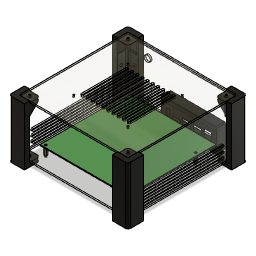
tp2_case_v1 (Autodesk Fusion 360 design; units mm, degrees)
Autodesk Fusion 360 part; units mm, degrees
sketch "Mini-ITX Board" plane through (0, 0, 0) normal (0, 1, 0) x (1, 0, 0)
  line L0 (0, 0) -> (170, 0)
  line L1 (170, 0) -> (170, 170)
  line L2 (170, 170) -> (0, 170)
  line L3 (0, 170) -> (0, 0)
  circle A0 centre (6.35, 159.84) radius 1.98
  circle A1 centre (6.35, 4.9) radius 1.98
  circle A2 centre (163.83, 4.9) radius 1.98
  circle A3 centre (163.83, 136.98) radius 1.98
  dimension "d1" = 170
  dimension "d2" = 170
  dimension "d3" = 3.96
  dimension "d4" = 10.16
  dimension "d5" = 6.35
  dimension "d6" = 3.96
  dimension "d7" = 154.94
  dimension "d8" = 6.35
  dimension "d9" = 3.96
  dimension "d10" = 157.48
  dimension "d11" = 154.94
  dimension "d12" = 3.96
  dimension "d13" = 22.86
  dimension "d14" = 157.48
  constraint horizontal L0
  constraint vertical L1
  constraint horizontal L2
  constraint vertical L3
  constraint coincident L0.start L3.end
  measures "d1" distance of L0.start L0.end
  measures "d2" distance of L0.start L2.end
  measures "d3" diameter of A0
  measures "d4" distance of L2 A0.centre
  measures "d5" distance of L3 A0.centre
  measures "d6" diameter of A1
  measures "d7" vertical distance of A0.centre A1.centre
  measures "d8" distance of L3 A1.centre
  measures "d9" diameter of A2
  measures "d10" horizontal distance of A1.centre A2.centre
  measures "d11" vertical distance of A0.centre A2.centre
  measures "d12" diameter of A3
  measures "d13" vertical distance of A0.centre A3.centre
  measures "d14" horizontal distance of A1.centre A3.centre
sketch "Base" plane through (0, 0, 0) normal (0, 1, 0) x (1, 0, 0)
  line L0 (-17, -20) -> (187, -20)
  line L1 (190, -17) -> (190, 187)
  line L2 (187, 190) -> (-17, 190)
  line L3 (-20, 187) -> (-20, -17)
  line L4 (170, 170) -> (0, 170)
  line L5 (0, 0) -> (170, 0)
  line L6 (170, 0) -> (170, 170)
  line L7 (0, 170) -> (0, 0)
  circle A0 centre (6.35, 159.84) radius 1.6
  circle A1 centre (6.35, 4.9) radius 1.6
  circle A2 centre (163.83, 4.9) radius 1.6
  circle A3 centre (163.83, 136.98) radius 1.6
  arc A4 (-17, 190) -> (-20, 187) centre (-17, 187) ccw
  arc A5 (190, 187) -> (187, 190) centre (187, 187) ccw
  arc A6 (187, -20) -> (190, -17) centre (187, -17) ccw
  arc A7 (-20, -17) -> (-17, -20) centre (-17, -17) ccw
  circle A8 centre (-10, -10) radius 1.6
  circle A9 centre (180, -10) radius 1.6
  circle A10 centre (180, 180) radius 1.6
  circle A11 centre (-10, 180) radius 1.6
  point P0 (6.35, 159.84)
  point P1 (163.83, 136.98)
  point P2 (163.83, 4.9)
  point P3 (6.35, 4.9)
  dimension "d15" = 20
  dimension "d16" = 20
  dimension "d17" = 20
  dimension "d18" = 20
  dimension "d19" = 3.2
  dimension "d20" = 3.2
  dimension "d21" = 3.2
  dimension "d22" = 3.2
  dimension "d57" = 3
  dimension "d88" = 3.2
  dimension "d89" = 10
  dimension "d90" = 10
  dimension "d91" = 3.2
  dimension "d92" = 10
  dimension "d93" = 10
  dimension "d94" = 3.2
  dimension "d95" = 10
  dimension "d96" = 10
  dimension "d97" = 3.2
  dimension "d98" = 10
  dimension "d99" = 10
  constraint horizontal L0
  constraint vertical L1
  constraint horizontal L2
  constraint vertical L3
  constraint coincident P0 A0.centre
  constraint coincident P3 A1.centre
  constraint coincident P2 A2.centre
  constraint coincident P1 A3.centre
  constraint tangent L2 A4
  constraint tangent L3 A4
  constraint tangent L1 A5
  constraint tangent L2 A5
  constraint equal A4 A5
  constraint tangent L0 A6
  constraint tangent L1 A6
  constraint equal A4 A6
  constraint tangent L0 A7
  constraint tangent L3 A7
  constraint equal A4 A7
  measures "d15" distance of L2 L4
  measures "d16" distance of L0 L5
  measures "d17" distance of L1 L6
  measures "d18" distance of L3 L7
  measures "d19" diameter of A0
  measures "d20" diameter of A1
  measures "d21" diameter of A2
  measures "d22" diameter of A3
  measures "d57" radius of A4
  measures "d88" diameter of A8
  measures "d89" distance of L0 A8.centre
  measures "d90" distance of L3 A8.centre
  measures "d91" diameter of A9
  measures "d92" distance of L1 A9.centre
  measures "d93" distance of L0 A9.centre
  measures "d94" diameter of A10
  measures "d95" distance of L1 A10.centre
  measures "d96" distance of L2 A10.centre
  measures "d97" diameter of A11
  measures "d98" distance of L2 A11.centre
  measures "d99" distance of L3 A11.centre
sketch "Top" plane through (0, 0, 0) normal (0, 1, 0) x (1, 0, 0)
  line L0 (-17, 190) -> (187, 190)
  line L1 (190, 187) -> (190, -17)
  line L2 (187, -20) -> (-17, -20)
  line L3 (-20, -17) -> (-20, 187)
  arc A0 (-17, 190) -> (-20, 187) centre (-17, 187) ccw
  arc A1 (190, 187) -> (187, 190) centre (187, 187) ccw
  arc A2 (187, -20) -> (190, -17) centre (187, -17) ccw
  arc A3 (-20, -17) -> (-17, -20) centre (-17, -17) ccw
  circle A4 centre (-10, -10) radius 1.6
  circle A5 centre (180, -10) radius 1.6
  circle A6 centre (180, 180) radius 1.6
  circle A7 centre (-10, 180) radius 1.6
  circle A8 centre (32.5, 137.5) radius 1.6
  circle A9 centre (137.5, 137.5) radius 1.6
  circle A10 centre (32.5, 32.5) radius 1.6
  circle A11 centre (137.5, 32.5) radius 1.6
  line L4 (35, 135) -> (135, 135)
  line L5 (135, 135) -> (135, 35)
  line L6 (135, 35) -> (35, 35)
  line L7 (35, 35) -> (35, 135)
  line L8 (39.5, 130) -> (40.5, 130)
  line L9 (42.5, 128) -> (42.5, 42)
  line L10 (40.5, 40) -> (39.5, 40)
  line L11 (37.5, 42) -> (37.5, 128)
  line L12 (49.5, 130) -> (50.5, 130)
  line L13 (52.5, 128) -> (52.5, 42)
  line L14 (47.5, 42) -> (47.5, 128)
  line L15 (50.5, 40) -> (49.5, 40)
  line L16 (59.5, 130) -> (60.5, 130)
  line L17 (62.5, 128) -> (62.5, 42)
  line L18 (57.5, 42) -> (57.5, 128)
  line L19 (60.5, 40) -> (59.5, 40)
  line L20 (69.5, 130) -> (70.5, 130)
  line L21 (72.5, 128) -> (72.5, 42)
  line L22 (67.5, 42) -> (67.5, 128)
  line L23 (70.5, 40) -> (69.5, 40)
  line L24 (79.5, 130) -> (80.5, 130)
  line L25 (82.5, 128) -> (82.5, 42)
  line L26 (77.5, 42) -> (77.5, 128)
  line L27 (80.5, 40) -> (79.5, 40)
  line L28 (89.5, 130) -> (90.5, 130)
  line L29 (92.5, 128) -> (92.5, 42)
  line L30 (87.5, 42) -> (87.5, 128)
  line L31 (90.5, 40) -> (89.5, 40)
  line L32 (99.5, 130) -> (100.5, 130)
  line L33 (102.5, 128) -> (102.5, 42)
  line L34 (97.5, 42) -> (97.5, 128)
  line L35 (100.5, 40) -> (99.5, 40)
  line L36 (109.5, 130) -> (110.5, 130)
  line L37 (112.5, 128) -> (112.5, 42)
  line L38 (107.5, 42) -> (107.5, 128)
  line L39 (110.5, 40) -> (109.5, 40)
  line L40 (119.5, 130) -> (120.5, 130)
  line L41 (122.5, 128) -> (122.5, 42)
  line L42 (117.5, 42) -> (117.5, 128)
  line L43 (120.5, 40) -> (119.5, 40)
  line L44 (129.5, 130) -> (130.5, 130)
  line L45 (132.5, 128) -> (132.5, 42)
  line L46 (127.5, 42) -> (127.5, 128)
  line L47 (130.5, 40) -> (129.5, 40)
  arc A12 (39.5, 130) -> (37.5, 128) centre (39.5, 128) ccw
  arc A13 (42.5, 128) -> (40.5, 130) centre (40.5, 128) ccw
  arc A14 (37.5, 42) -> (39.5, 40) centre (39.5, 42) ccw
  arc A15 (40.5, 40) -> (42.5, 42) centre (40.5, 42) ccw
  arc A16 (47.5, 42) -> (49.5, 40) centre (49.5, 42) ccw
  arc A17 (50.5, 40) -> (52.5, 42) centre (50.5, 42) ccw
  arc A18 (49.5, 130) -> (47.5, 128) centre (49.5, 128) ccw
  arc A19 (52.5, 128) -> (50.5, 130) centre (50.5, 128) ccw
  arc A20 (57.5, 42) -> (59.5, 40) centre (59.5, 42) ccw
  arc A21 (60.5, 40) -> (62.5, 42) centre (60.5, 42) ccw
  arc A22 (59.5, 130) -> (57.5, 128) centre (59.5, 128) ccw
  arc A23 (62.5, 128) -> (60.5, 130) centre (60.5, 128) ccw
  arc A24 (69.5, 130) -> (67.5, 128) centre (69.5, 128) ccw
  arc A25 (72.5, 128) -> (70.5, 130) centre (70.5, 128) ccw
  arc A26 (67.5, 42) -> (69.5, 40) centre (69.5, 42) ccw
  arc A27 (70.5, 40) -> (72.5, 42) centre (70.5, 42) ccw
  arc A28 (77.5, 42) -> (79.5, 40) centre (79.5, 42) ccw
  arc A29 (80.5, 40) -> (82.5, 42) centre (80.5, 42) ccw
  arc A30 (82.5, 128) -> (80.5, 130) centre (80.5, 128) ccw
  arc A31 (79.5, 130) -> (77.5, 128) centre (79.5, 128) ccw
  arc A32 (89.5, 130) -> (87.5, 128) centre (89.5, 128) ccw
  arc A33 (92.5, 128) -> (90.5, 130) centre (90.5, 128) ccw
  arc A34 (87.5, 42) -> (89.5, 40) centre (89.5, 42) ccw
  arc A35 (90.5, 40) -> (92.5, 42) centre (90.5, 42) ccw
  arc A36 (97.5, 42) -> (99.5, 40) centre (99.5, 42) ccw
  arc A37 (100.5, 40) -> (102.5, 42) centre (100.5, 42) ccw
  arc A38 (102.5, 128) -> (100.5, 130) centre (100.5, 128) ccw
  arc A39 (99.5, 130) -> (97.5, 128) centre (99.5, 128) ccw
  arc A40 (109.5, 130) -> (107.5, 128) centre (109.5, 128) ccw
  arc A41 (112.5, 128) -> (110.5, 130) centre (110.5, 128) ccw
  arc A42 (107.5, 42) -> (109.5, 40) centre (109.5, 42) ccw
  arc A43 (110.5, 40) -> (112.5, 42) centre (110.5, 42) ccw
  arc A44 (117.5, 42) -> (119.5, 40) centre (119.5, 42) ccw
  arc A45 (120.5, 40) -> (122.5, 42) centre (120.5, 42) ccw
  arc A46 (122.5, 128) -> (120.5, 130) centre (120.5, 128) ccw
  arc A47 (119.5, 130) -> (117.5, 128) centre (119.5, 128) ccw
  arc A48 (129.5, 130) -> (127.5, 128) centre (129.5, 128) ccw
  arc A49 (132.5, 128) -> (130.5, 130) centre (130.5, 128) ccw
  arc A50 (130.5, 40) -> (132.5, 42) centre (130.5, 42) ccw
  arc A51 (127.5, 42) -> (129.5, 40) centre (129.5, 42) ccw
  point P0 (-20, 190)
  point P1 (190, -20)
  point P2 (37.5, 130)
  point P3 (42.5, 130)
  point P4 (37.5, 40)
  dimension "d59" = 3
  dimension "d146" = 3.2
  dimension "d147" = 3.2
  dimension "d148" = 3.2
  dimension "d149" = 3.2
  dimension "d150" = 52.5
  dimension "d151" = 52.5
  dimension "d152" = 52.5
  dimension "d153" = 52.5
  dimension "d154" = 52.5
  dimension "d155" = 52.5
  dimension "d156" = 105
  dimension "d157" = 52.5
  dimension "d158" = 52.5
  dimension "d159" = 105
  dimension "d160" = 100
  dimension "d161" = 100
  dimension "d162" = 2.5
  dimension "d163" = 2.5
  dimension "d164" = 5
  dimension "d165" = 90
  dimension "d166" = 2.5
  dimension "d167" = 5
  dimension "d172" = 2
  constraint horizontal L0
  constraint vertical L1
  constraint horizontal L2
  constraint vertical L3
  constraint tangent L0 A0
  constraint tangent L3 A0
  constraint tangent L0 A1
  constraint tangent L1 A1
  constraint equal A0 A1
  constraint tangent L1 A2
  constraint tangent L2 A2
  constraint equal A0 A2
  constraint tangent L2 A3
  constraint tangent L3 A3
  constraint equal A0 A3
  constraint horizontal L4
  constraint vertical L5
  constraint horizontal L6
  constraint vertical L7
  constraint horizontal L8
  constraint vertical L9
  constraint horizontal L10
  constraint vertical L11
  constraint coincident P2 L8
  constraint coincident P2 L11
  constraint tangent L8 A12
  constraint tangent L11 A12
  constraint coincident P3 L8
  constraint coincident P3 L9
  constraint tangent L8 A13
  constraint tangent L9 A13
  constraint equal A12 A13
  constraint coincident P4 L10
  constraint coincident P4 L11
  constraint tangent L10 A14
  constraint tangent L11 A14
  constraint equal A12 A14
  constraint tangent L9 A15
  constraint tangent L10 A15
  constraint equal A12 A15
  constraint tangent L14 A16
  constraint tangent L15 A16
  constraint equal A12 A16
  constraint tangent L13 A17
  constraint tangent L15 A17
  constraint equal A12 A17
  constraint tangent L12 A18
  constraint tangent L14 A18
  constraint equal A12 A18
  constraint tangent L12 A19
  constraint tangent L13 A19
  constraint equal A12 A19
  constraint tangent L18 A20
  constraint tangent L19 A20
  constraint equal A12 A20
  constraint tangent L17 A21
  constraint tangent L19 A21
  constraint equal A12 A21
  constraint tangent L16 A22
  constraint tangent L18 A22
  constraint equal A12 A22
  constraint tangent L16 A23
  constraint tangent L17 A23
  constraint equal A12 A23
  constraint tangent L20 A24
  constraint tangent L22 A24
  constraint equal A12 A24
  constraint tangent L20 A25
  constraint tangent L21 A25
  constraint equal A12 A25
  constraint tangent L22 A26
  constraint tangent L23 A26
  constraint equal A12 A26
  constraint tangent L21 A27
  constraint tangent L23 A27
  constraint equal A12 A27
  constraint tangent L26 A28
  constraint tangent L27 A28
  constraint equal A12 A28
  constraint tangent L25 A29
  constraint tangent L27 A29
  constraint equal A12 A29
  constraint tangent L24 A30
  constraint tangent L25 A30
  constraint equal A12 A30
  constraint tangent L24 A31
  constraint tangent L26 A31
  constraint equal A12 A31
  constraint tangent L28 A32
  constraint tangent L30 A32
  constraint equal A12 A32
  constraint tangent L28 A33
  constraint tangent L29 A33
  constraint equal A12 A33
  constraint tangent L30 A34
  constraint tangent L31 A34
  constraint equal A12 A34
  constraint tangent L29 A35
  constraint tangent L31 A35
  constraint equal A12 A35
  constraint tangent L34 A36
  constraint tangent L35 A36
  constraint equal A12 A36
  constraint tangent L33 A37
  constraint tangent L35 A37
  constraint equal A12 A37
  constraint tangent L32 A38
  constraint tangent L33 A38
  constraint equal A12 A38
  constraint tangent L32 A39
  constraint tangent L34 A39
  constraint equal A12 A39
  constraint tangent L36 A40
  constraint tangent L38 A40
  constraint equal A12 A40
  constraint tangent L36 A41
  constraint tangent L37 A41
  constraint equal A12 A41
  constraint tangent L38 A42
  constraint tangent L39 A42
  constraint equal A12 A42
  constraint tangent L37 A43
  constraint tangent L39 A43
  constraint equal A12 A43
  constraint tangent L42 A44
  constraint tangent L43 A44
  constraint equal A12 A44
  constraint tangent L41 A45
  constraint tangent L43 A45
  constraint equal A12 A45
  constraint tangent L40 A46
  constraint tangent L41 A46
  constraint equal A12 A46
  constraint tangent L40 A47
  constraint tangent L42 A47
  constraint equal A12 A47
  constraint tangent L44 A48
  constraint tangent L46 A48
  constraint equal A12 A48
  constraint tangent L44 A49
  constraint tangent L45 A49
  constraint equal A12 A49
  constraint tangent L45 A50
  constraint tangent L47 A50
  constraint equal A12 A50
  constraint tangent L46 A51
  constraint tangent L47 A51
  constraint equal A12 A51
  measures "d59" radius of A0
  measures "d146" diameter of A8
  measures "d147" diameter of A9
  measures "d148" diameter of A10
  measures "d149" diameter of A11
  measures "d150" distance of L0 A9.centre
  measures "d151" distance of L1 A9.centre
  measures "d152" distance of L1 A11.centre
  measures "d153" distance of L2 A11.centre
  measures "d154" distance of L2 A10.centre
  measures "d155" distance of L3 A10.centre
  measures "d156" distance of A10.centre A11.centre
  measures "d157" distance of L0 A8.centre
  measures "d158" distance of L3 A8.centre
  measures "d159" distance of A8.centre A10.centre
  measures "d160" distance of L4.start L4.end
  measures "d161" distance of L4.start L6.end
  measures "d162" distance of A10.centre L7
  measures "d163" distance of A8.centre L4
  measures "d164" distance of P2 P3
  measures "d165" distance of P2 P4
  measures "d166" distance of L7 L11
  measures "d167" distance of L4 L8
  measures "d172" radius of A12
sketch "Leg" plane through (0, 0, 0) normal (0, 1, 0) x (1, 0, 0)
  line L0 (-10, -10) -> (-30, -10)
  line L1 (-30, -10) -> (-30, -25)
  line L2 (-25, -30) -> (-10, -30)
  line L3 (-10, -30) -> (-10, -10)
  line L4 (-20, -17) -> (-20, 187)
  line L5 (187, -20) -> (-17, -20)
  line L6 (-17, -20) -> (187, -20)
  line L7 (-20, 187) -> (-20, -17)
  line L8 (-30, -30) -> (0, -30)
  line L9 (0, -30) -> (0, -5)
  line L10 (-5, 0) -> (-30, 0)
  line L11 (-30, 0) -> (-30, -30)
  arc A0 (-30, -25) -> (-25, -30) centre (-25, -25) ccw
  arc A1 (0, -5) -> (-5, 0) centre (-5, -5) ccw
  line L12 (-20, -20.25) -> (0, -20.25)
  line L13 (0, -20.25) -> (0, 0)
  line L14 (0, 0) -> (-20.25, 0)
  line L15 (-20.25, 0) -> (-20.25, -20)
  line L16 (-20.25, -20) -> (-20.25, -20.25)
  line L17 (-20.25, -20.25) -> (-20, -20.25)
  dimension "d23" = 10
  dimension "d24" = 10
  dimension "d25" = 10
  dimension "d26" = 10
  dimension "d48" = 5
  dimension "d49" = 5
  dimension "d55" = 0.25
  dimension "d56" = 0.25
  constraint horizontal L0
  constraint vertical L1
  constraint horizontal L2
  constraint vertical L3
  constraint horizontal L8
  constraint vertical L9
  constraint horizontal L10
  constraint vertical L11
  constraint coincident L8.start L2
  constraint coincident L8.start L1
  constraint tangent L2 A0
  constraint tangent L1 A0
  constraint tangent L9 A1
  constraint tangent L10 A1
  constraint horizontal L12
  constraint vertical L13
  constraint horizontal L14
  constraint vertical L15
  constraint coincident L13.end L14.start
  constraint perpendicular L12 L16
  constraint perpendicular L16 L17
  measures "d23" distance of L3 L4
  measures "d24" distance of L0 L5
  measures "d25" distance of L2 L6
  measures "d26" distance of L1 L7
  measures "d48" radius of A0
  measures "d49" radius of A1
  measures "d55" distance of L5 L12
  measures "d56" distance of L4 L15
extrude "Extrude1" add sketch "Mini-ITX Board" along normal blind 1.7 makes body 1
sketch "Standoffs" plane through (0, 0, 0) normal (0, 1, 0) x (1, 0, 0)
  line L0 (8.85, 161.2834) -> (6.35, 162.7268)
  line L1 (6.35, 162.7268) -> (3.85, 161.2834)
  line L2 (3.85, 161.2834) -> (3.85, 158.3966)
  line L3 (3.85, 158.3966) -> (6.35, 156.9532)
  line L4 (6.35, 156.9532) -> (8.85, 158.3966)
  line L5 (8.85, 158.3966) -> (8.85, 161.2834)
  line L6 (161.33, 135.5366) -> (163.83, 134.0932)
  line L7 (163.83, 134.0932) -> (166.33, 135.5366)
  line L8 (166.33, 135.5366) -> (166.33, 138.4234)
  line L9 (166.33, 138.4234) -> (163.83, 139.8668)
  line L10 (163.83, 139.8668) -> (161.33, 138.4234)
  line L11 (161.33, 138.4234) -> (161.33, 135.5366)
  line L12 (8.85, 6.3434) -> (6.35, 7.7868)
  line L13 (6.35, 7.7868) -> (3.85, 6.3434)
  line L14 (3.85, 6.3434) -> (3.85, 3.4566)
  line L15 (3.85, 3.4566) -> (6.35, 2.0132)
  line L16 (6.35, 2.0132) -> (8.85, 3.4566)
  line L17 (8.85, 3.4566) -> (8.85, 6.3434)
  line L18 (161.33, 3.4566) -> (163.83, 2.0132)
  line L19 (163.83, 2.0132) -> (166.33, 3.4566)
  line L20 (166.33, 3.4566) -> (166.33, 6.3434)
  line L21 (166.33, 6.3434) -> (163.83, 7.7868)
  line L22 (163.83, 7.7868) -> (161.33, 6.3434)
  line L23 (161.33, 6.3434) -> (161.33, 3.4566)
  point P0 (163.83, 136.98)
  point P1 (6.35, 159.84)
  point P2 (6.35, 4.9)
  point P3 (163.83, 4.9)
  point P4 (6.35, 159.84)
  point P5 (163.83, 136.98)
  point P6 (6.35, 4.9)
  point P7 (163.83, 4.9)
  dimension "d29" = 2.5
  dimension "d30" = 2.5
  dimension "d31" = 2.5
  dimension "d32" = 2.5
  constraint coincident P4 P1
  constraint coincident P5 P0
  constraint coincident P6 P2
  constraint coincident P7 P3
  measures "d29" distance of P4 L5
  measures "d30" distance of P5 L11
  measures "d31" distance of P6 L17
  measures "d32" distance of P7 L23
extrude "Extrude2" add sketch "Standoffs" against normal blind 15 separate body makes body 2 at (161.33, -5, -137.4611) makes body 3 at (162.1633, -5, -2.9755) makes body 4 at (8.85, -10, -159.3589) makes body 5 at (8.85, -5, -4.4189)
extrude "Extrude3" add sketch "Base" against normal blind 3 from surface at -15 separate body contours L0 L1 L2 L3 A4 A5 A6 A7 | L4 L5 L6 L7 makes body 6
extrude "Extrude4" add sketch "Leg" against normal blind 8 from surface at -18 separate body contours L0 L3 L12 L15 L16 L17 | L0 L3 L4 L5 L6 L7 L9 L10 A1 L13 L14 | L0 L4 L7 L10 L14 L15 | L3 L5 L6 L9 L12 L13 | L0 L1 L2 L3 L8 L11 A0 L12 L15 L16 L17 | L0 L10 L11 L15 | L3 L8 L9 L12 makes body 7
extrude "Extrude5" add sketch "Leg" along normal blind 102.7 from surface at -18 contours L0 L1 L2 L3 L8 L11 A0 L12 L15 L16 L17 | L0 L10 L11 L15 | L3 L8 L9 L12 bodies 7
extrude "Extrude7" add sketch "Leg" against normal blind 5 from surface at 81.7 contours L0 L3 L12 L15 L16 L17 | L0 L3 L4 L5 L6 L7 L9 L10 A1 L13 L14 | L0 L4 L7 L10 L14 L15 | L3 L5 L6 L9 L12 L13 | L0 L1 L2 L3 L8 L11 A0 L12 L15 L16 L17 | L0 L10 L11 L15 | L3 L8 L9 L12 bodies 7
chamfer "Chamfer1" distance 18 angle 45 2 edges at (-20.25, 76.7, 10.125) (-10.125, 76.7, 20.25) on bodies 7
fillet "Fillet1" radius 3 1 edges at (-20.25, 83.2, 20.25) on bodies 7
extrude "Extrude8" add sketch "Top" along normal blind 3 from surface at 81.7 separate body contours L0 L1 L2 L3 A0 A1 A2 A3 | L4 L5 L6 L7 makes body 8
sketch "Leg Holes 1" plane through (0, 0, 0) normal (0, 1, 0) x (1, 0, 0)
  circle A0 centre (-10, -10) radius 1.6
  circle A1 centre (-10, -10) radius 2.65
  point P0 (-10, -10)
  dimension "d100" = 3.2
  dimension "d101" = 5.3
  constraint coincident P0 A0.centre
  measures "d100" diameter of A0
  measures "d101" diameter of A1
sketch "Leg Holes 2" plane through (0, 0, 20.25) normal (0, 0, -1) x (-1, 0, 0)
  line L0 (20.25, 58.7) -> (0, 58.7)
  line L1 (0, 58.7) -> (0, -18)
  line L2 (0, -18) -> (20.25, -18)
  line L3 (20.25, -18) -> (20.25, 58.7)
  circle A0 centre (7, 10.5) radius 1.6
  circle A1 centre (7, 36) radius 1.6
  circle A2 centre (7, 36) radius 2.65
  circle A3 centre (7, 10.5) radius 2.65
  dimension "d102" = 3.2
  dimension "d103" = 28.5
  dimension "d104" = 7
  dimension "d105" = 3.2
  dimension "d106" = 7
  dimension "d107" = 25.5
  dimension "d108" = 5.3
  dimension "d109" = 5.3
  constraint concentric A1 A2
  constraint concentric A0 A3
  measures "d102" diameter of A0
  measures "d103" distance of L2 A0.centre
  measures "d104" distance of L1 A0.centre
  measures "d105" diameter of A1
  measures "d106" distance of L1 A1.centre
  measures "d107" distance of A0.centre A1.centre
  measures "d108" diameter of A2
  measures "d109" diameter of A3
sketch "Leg Holes 3" plane through (-20.25, 0, 0) normal (1, 0, 0) x (0, 0, -1)
  line L0 (0, 58.7) -> (-20.25, 58.7)
  line L1 (-20.25, 58.7) -> (-20.25, -18)
  line L2 (-20.25, -18) -> (0, -18)
  line L3 (0, -18) -> (0, 58.7)
  circle A0 centre (-7, 10.5) radius 1.6
  circle A1 centre (-7, 36) radius 1.6
  circle A2 centre (-7, 36) radius 2.65
  circle A3 centre (-7, 10.5) radius 2.65
  dimension "d110" = 3.2
  dimension "d111" = 7
  dimension "d112" = 28.5
  dimension "d113" = 3.2
  dimension "d114" = 25.5
  dimension "d115" = 7
  dimension "d116" = 5.3
  dimension "d117" = 5.3
  constraint concentric A1 A2
  constraint concentric A0 A3
  measures "d110" diameter of A0
  measures "d111" distance of L3 A0.centre
  measures "d112" distance of L2 A0.centre
  measures "d113" diameter of A1
  measures "d114" vertical distance of A0.centre A1.centre
  measures "d115" distance of L3 A1.centre
  measures "d116" diameter of A2
  measures "d117" diameter of A3
extrude "Extrude10" cut sketch "Leg Holes 2" against normal blind 6.3 contours A0 | A1 bodies 7
extrude "Extrude11" cut sketch "Leg Holes 3" against normal blind 6.3 contours A0 | A1 bodies 7
extrude "Extrude12" cut sketch "Leg Holes 3" against normal blind 3.8 contours A2 | A3 bodies 7
extrude "Extrude13" cut sketch "Leg Holes 2" against normal blind 3.8 contours A2 | A3 bodies 7
extrude "Extrude14" cut sketch "Leg Holes 1" against normal blind 6.3 from surface at -18 contours A0 bodies 7
extrude "Extrude15" cut sketch "Leg Holes 1" against normal blind 3.8 from surface at -18 bodies 7
extrude "Extrude16" cut sketch "Leg Holes 1" against normal blind 6.3 from surface at 81.7 contours A0 bodies 7
extrude "Extrude17" cut sketch "Leg Holes 1" against normal blind 3.8 from surface at 81.7 bodies 7
copy_body "CopyPasteBodies1" bodies 7 makes body 9
move_body "Move1" bodies 9 to x (1, 0, 0) y (0, 1, 0) z (0, 0, 1) at (240, 0, 0)
move_body "Move2" bodies 9 to x (0, 0, -1) y (0, 1, 0) z (1, 0, 0) at (210, 0, 270)
move_body "Move3" bodies 9 to x (1, 0, 0) y (0, 1, 0) z (0, 0, 1) at (-40, 0, -30)
copy_body "CopyPasteBodies2" bodies 9 makes body 10
move_body "Move4" bodies 10 to x (1, 0, 0) y (0, 1, 0) z (0, 0, 1) at (0, 0, -250)
move_body "Move5" bodies 10 to x (0, 0, -1) y (0, 1, 0) z (1, 0, 0) at (390, 0, -50)
move_body "Move6" bodies 10 to x (1, 0, 0) y (0, 1, 0) z (0, 0, 1) at (30, 0, 50)
copy_body "CopyPasteBodies3" bodies 10 makes body 11
move_body "Move7" bodies 11 to x (1, 0, 0) y (0, 1, 0) z (0, 0, 1) at (-240, 0, 0)
move_body "Move8" bodies 11 to x (0, 0, -1) y (0, 1, 0) z (1, 0, 0) at (130, 0, -210)
move_body "Move9" bodies 11 to x (1, 0, 0) y (0, 1, 0) z (0, 0, 1) at (40, 0, -30)
sketch "Front/Back" plane through (0, 0, 0) normal (0, 0, 1) x (1, 0, 0)
  line L0 (-20.25, 58.7) -> (0, 58.7)
  line L1 (-17, -15) -> (187, -15)
  line L2 (-15.25, -15) -> (185.25, -15)
  line L3 (185.25, -15) -> (185.25, 57.7)
  line L4 (185.25, 57.7) -> (-15.25, 57.7)
  line L5 (-15.25, 57.7) -> (-15.25, -15)
  line L6 (190.25, -18) -> (190.25, 58.7)
  line L7 (-20.25, -18) -> (-20.25, 58.7)
  line L8 (0, -18) -> (0, 58.7)
  line L9 (187, 81.7) -> (-17, 81.7)
  line L10 (170, -18) -> (170, 58.7)
  line L11 (170, 81.7) -> (170, 73.95)
  line L12 (0, 57.7) -> (170, 57.7)
  line L13 (170, 57.7) -> (170, 81.7)
  line L14 (170, 81.7) -> (0, 81.7)
  line L15 (0, 81.7) -> (0, 57.7)
  line L16 (7, -5) -> (163, -5)
  line L17 (165, -7) -> (165, -8)
  line L18 (163, -10) -> (7, -10)
  line L19 (5, -8) -> (5, -7)
  line L20 (7, 5) -> (163, 5)
  line L21 (5, 2) -> (5, 3)
  line L22 (163, 0) -> (7, 0)
  line L23 (165, 3) -> (165, 2)
  line L24 (7, 15) -> (163, 15)
  line L25 (5, 12) -> (5, 13)
  line L26 (163, 10) -> (7, 10)
  line L27 (165, 13) -> (165, 12)
  arc A0 (7, 15) -> (5, 13) centre (7, 13) ccw
  arc A1 (5, 12) -> (7, 10) centre (7, 12) ccw
  arc A2 (165, 13) -> (163, 15) centre (163, 13) ccw
  arc A3 (163, 10) -> (165, 12) centre (163, 12) ccw
  arc A4 (165, 3) -> (163, 5) centre (163, 3) ccw
  arc A5 (163, 0) -> (165, 2) centre (163, 2) ccw
  arc A6 (7, 5) -> (5, 3) centre (7, 3) ccw
  arc A7 (5, 2) -> (7, 0) centre (7, 2) ccw
  arc A8 (7, -5) -> (5, -7) centre (7, -7) ccw
  arc A9 (5, -8) -> (7, -10) centre (7, -8) ccw
  arc A10 (165, -7) -> (163, -5) centre (163, -7) ccw
  arc A11 (163, -10) -> (165, -8) centre (163, -8) ccw
  circle A12 centre (177, 36) radius 1.6
  circle A13 centre (177, 10.5) radius 1.6
  circle A14 centre (-7, 36) radius 1.6
  circle A15 centre (-7, 10.5) radius 1.6
  point P0 (5, -5)
  point P1 (5, -10)
  dimension "d138" = 5
  dimension "d139" = 5
  dimension "d140" = 1
  dimension "d173" = 5
  dimension "d174" = 5
  dimension "d175" = 5
  dimension "d176" = 5
  dimension "d181" = 2
  constraint horizontal L2
  constraint vertical L3
  constraint horizontal L4
  constraint vertical L5
  constraint coincident L1 L2.start
  constraint horizontal L12
  constraint vertical L13
  constraint horizontal L14
  constraint vertical L15
  constraint coincident L11.start L13.end
  constraint coincident L4 L12.start
  constraint coincident L8 L12.start
  constraint horizontal L16
  constraint vertical L17
  constraint horizontal L18
  constraint vertical L19
  constraint tangent L24 A0
  constraint tangent L25 A0
  constraint tangent L25 A1
  constraint tangent L26 A1
  constraint equal A0 A1
  constraint tangent L24 A2
  constraint tangent L27 A2
  constraint equal A0 A2
  constraint tangent L26 A3
  constraint tangent L27 A3
  constraint equal A0 A3
  constraint tangent L20 A4
  constraint tangent L23 A4
  constraint equal A0 A4
  constraint tangent L22 A5
  constraint tangent L23 A5
  constraint equal A0 A5
  constraint tangent L20 A6
  constraint tangent L21 A6
  constraint equal A0 A6
  constraint tangent L21 A7
  constraint tangent L22 A7
  constraint equal A0 A7
  constraint coincident P0 L16
  constraint coincident P0 L19
  constraint tangent L16 A8
  constraint tangent L19 A8
  constraint equal A0 A8
  constraint coincident P1 L18
  constraint coincident P1 L19
  constraint tangent L18 A9
  constraint tangent L19 A9
  constraint equal A0 A9
  constraint tangent L16 A10
  constraint tangent L17 A10
  constraint equal A0 A10
  constraint tangent L17 A11
  constraint tangent L18 A11
  constraint equal A0 A11
  measures "d138" distance of L5 L7
  measures "d139" distance of L3 L6
  measures "d140" distance of L0 L4
  measures "d173" distance of P0 P1
  measures "d174" distance of L8 L19
  measures "d175" distance of L10 L17
  measures "d176" distance of L2 L18
  measures "d181" radius of A0
extrude "Extrude1'" add sketch "Front/Back" against normal blind 3 from surface at 20.25 separate body contours L1 L2 L4 L5 L8 | L1 L2 L4 L8 L10 L12 | L1 L2 L3 L4 L10 | L4 L8 L9 L10 L11 L12 L13 L14 L15 | L16 L17 L18 L19 A8 A9 A10 A11 | L20 L21 L22 L23 A4 A5 A6 A7 | L24 L25 L26 L27 A0 A1 A2 A3 | A12 | A13 | A14 | A15 makes body 12 in component "Component"
extrude "Extrude2'" cut 4 faces at (177.5274, 11.146, 26.55) (177.4805, 35.7686, 26.55) (-6.609, 35.6372, 26.55) (-6.871, 10.9516, 26.55) along direction (0, 0, -1) blind 20 on bodies 7 9 bodies 12 in component "Component"
extrude "Extrude18" add sketch "Front/Back" against normal blind 3 from surface at 20.25 separate body contours L1 L2 L4 L5 L8 | L1 L2 L4 L8 L10 L12 | L1 L2 L3 L4 L10 | L4 L8 L9 L10 L11 L12 L13 L14 L15 | A12 | A13 | A14 | A15 makes body 13
move_body "Move10" bodies 13 to x (1, 0, 0) y (0, 1, 0) z (0, 0, 1) at (310, 0, -50)
move_body "Move11" bodies 13 to x (0, 0, -1) y (0, 1, 0) z (1, 0, 0) at (528, 0, 462.5)
move_body "Move12" bodies 13 to x (1, 0, 0) y (0, 1, 0) z (0, 0, 1) at (-310, 0, -150)
move_body "Move13" bodies 13 to x (1, 0, 0) y (0, 1, 0) z (0, 0, 1) at (0, 0, -2.5)
move_body "Move14" bodies 13 to x (1, 0, 0) y (0, 1, 0) z (0, 0, 1) at (2, 0, 0)
copy_body "CopyPasteBodies4" bodies 13 makes body 14
move_body "Move15" bodies 14 to x (1, 0, 0) y (0, 1, 0) z (0, 0, 1) at (-210, 0, 0)
sketch "Back Plate" plane through (0, 0, 0) normal (0, 0, 1) x (1, 0, 0)
  line L0 (170, 81.7) -> (170, 57.7)
  line L1 (170, 57.7) -> (185.25, 57.7)
  line L2 (185.25, 57.7) -> (185.25, -15)
  line L3 (185.25, -15) -> (-15.25, -15)
  line L4 (-15.25, -15) -> (-15.25, 57.7)
  line L5 (-15.25, 57.7) -> (0, 57.7)
  line L6 (0, 57.7) -> (0, 81.7)
  line L7 (0, 81.7) -> (170, 81.7)
  circle A0 centre (20, -7) radius 3.9
  circle A1 centre (177, 36) radius 1.6
  circle A2 centre (177, 10.5) radius 1.6
  circle A3 centre (-7, 36) radius 1.6
  circle A4 centre (-7, 10.5) radius 1.6
  circle A5 centre (20, 61.7) radius 6
  line L8 (170, 23) -> (65, 23)
  line L9 (65, 23) -> (65, -7)
  line L10 (65, -7) -> (170, -7)
  line L11 (170, -7) -> (170, 23)
  circle A6 centre (145, -11) radius 1.6
  circle A7 centre (90, -11) radius 1.6
  circle A8 centre (145, 27) radius 1.6
  circle A9 centre (90, 27) radius 1.6
  point P0 (0, 57.7)
  point P1 (0, 81.7)
  point P2 (170, 81.7)
  point P3 (170, 57.7)
  point P4 (185.25, 57.7)
  point P5 (185.25, -15)
  point P6 (-15.25, -15)
  point P7 (-15.25, 57.7)
  point P8 (177, 36)
  point P9 (177, 10.5)
  point P10 (-7, 36)
  point P11 (-7, 10.5)
  dimension "d201" = 7.8
  dimension "d202" = 20
  dimension "d203" = 8
  dimension "d204" = 3.2
  dimension "d205" = 3.2
  dimension "d206" = 3.2
  dimension "d207" = 3.2
  dimension "d208" = 12
  dimension "d209" = 20
  dimension "d210" = 20
  dimension "d211" = 38
  dimension "d212" = 8
  dimension "d213" = 15.25
  dimension "d214" = 105
  dimension "d215" = 3.2
  dimension "d216" = 3.2
  dimension "d217" = 3.2
  dimension "d218" = 3.2
  dimension "d219" = 25
  dimension "d220" = 25
  dimension "d221" = 25
  dimension "d222" = 25
  dimension "d223" = 4
  dimension "d224" = 4
  dimension "d225" = 4
  dimension "d226" = 4
  constraint coincident P2 L0.start
  constraint coincident P3 L0.end
  constraint coincident P4 L1.end
  constraint coincident P5 L2.end
  constraint coincident P6 L3.end
  constraint coincident P7 L4.end
  constraint coincident P0 L5.end
  constraint coincident P1 L6.end
  constraint coincident P8 A1.centre
  constraint coincident P9 A2.centre
  constraint coincident P10 A3.centre
  constraint coincident P11 A4.centre
  constraint horizontal L8
  constraint vertical L9
  constraint horizontal L10
  constraint vertical L11
  measures "d201" diameter of A0
  measures "d202" distance of L6 A0.centre
  measures "d203" distance of L3 A0.centre
  measures "d204" diameter of A1
  measures "d205" diameter of A2
  measures "d206" diameter of A3
  measures "d207" diameter of A4
  measures "d208" diameter of A5
  measures "d209" distance of L6 A5.centre
  measures "d210" distance of L7 A5.centre
  measures "d211" distance of L3 L8
  measures "d212" distance of L3 L10
  measures "d213" distance of L2 L11
  measures "d214" distance of L9 L11
  measures "d215" diameter of A6
  measures "d216" diameter of A7
  measures "d217" diameter of A8
  measures "d218" diameter of A9
  measures "d219" distance of L9 A9.centre
  measures "d220" distance of L11 A8.centre
  measures "d221" distance of L9 A7.centre
  measures "d222" distance of L11 A6.centre
  measures "d223" distance of L10 A6.centre
  measures "d224" distance of L10 A7.centre
  measures "d225" distance of L8 A8.centre
  measures "d226" distance of L8 A9.centre
extrude "Extrude19" add sketch "Back Plate" along normal blind 3 from surface at -190.25 separate body makes body 15
sketch "IO Plate" plane through (0, 0, 0) normal (0, 0, 1) x (1, 0, 0)
  line L0 (170, 23) -> (65, 23)
  line L1 (170, -7) -> (170, 23)
  line L2 (65, 23) -> (65, -7)
  line L3 (65, -7) -> (170, -7)
  line L4 (185.25, -15) -> (-15.25, -15)
  line L5 (171.2, 31) -> (63.8, 31)
  line L6 (63.8, 31) -> (63.8, -15)
  line L7 (63.8, -15) -> (171.2, -15)
  line L8 (171.2, -15) -> (171.2, 31)
  circle A0 centre (145, 27) radius 2.65
  circle A1 centre (90, 27) radius 2.65
  circle A2 centre (90, -11) radius 2.65
  circle A3 centre (145, -11) radius 2.65
  line L9 (170, 1.7) -> (0, 1.7)
  line L10 (161, 1.7) -> (146.5, 1.7)
  line L11 (146.5, 1.7) -> (146.5, 16.95)
  line L12 (146.5, 16.95) -> (161, 16.95)
  line L13 (161, 16.95) -> (161, 1.7)
  line L14 (141.65, 1.7) -> (125.65, 1.7)
  line L15 (125.65, 1.7) -> (125.65, 14.7)
  line L16 (125.65, 14.7) -> (141.65, 14.7)
  line L17 (141.65, 14.7) -> (141.65, 1.7)
  line L18 (121.05, 1.7) -> (105.05, 1.7)
  line L19 (105.05, 1.7) -> (105.05, 14.7)
  line L20 (105.05, 14.7) -> (121.05, 14.7)
  line L21 (121.05, 14.7) -> (121.05, 1.7)
  line L22 (100.45, 1.7) -> (85.45, 1.7)
  line L23 (85.45, 1.7) -> (85.45, 7.7)
  line L24 (85.45, 7.7) -> (100.45, 7.7)
  line L25 (100.45, 7.7) -> (100.45, 1.7)
  line L26 (80.1, 1.7) -> (74.1, 1.7)
  line L27 (74.1, 1.7) -> (74.1, 15.45)
  line L28 (74.1, 15.45) -> (80.1, 15.45)
  line L29 (80.1, 15.45) -> (80.1, 1.7)
  point P0 (145, 27)
  point P1 (90, 27)
  point P2 (90, -11)
  point P3 (145, -11)
  dimension "d230" = 1.2
  dimension "d231" = 1.2
  dimension "d232" = 8
  dimension "d233" = 5.3
  dimension "d234" = 5.3
  dimension "d235" = 5.3
  dimension "d236" = 5.3
  dimension "d237" = 15.25
  dimension "d238" = 9
  dimension "d239" = 14.5
  dimension "d240" = 13
  dimension "d241" = 4.85
  dimension "d242" = 16
  dimension "d243" = 16
  dimension "d244" = 13
  dimension "d245" = 4.6
  dimension "d246" = 15
  dimension "d247" = 6
  dimension "d248" = 4.6
  dimension "d249" = 6
  dimension "d250" = 13.75
  dimension "d251" = 5.35
  constraint horizontal L5
  constraint vertical L6
  constraint horizontal L7
  constraint vertical L8
  constraint coincident L4 L6.end
  constraint coincident P0 A0.centre
  constraint coincident P1 A1.centre
  constraint coincident P2 A2.centre
  constraint coincident P3 A3.centre
  constraint horizontal L10
  constraint vertical L11
  constraint horizontal L12
  constraint vertical L13
  constraint coincident L9 L10.start
  constraint horizontal L14
  constraint vertical L15
  constraint horizontal L16
  constraint vertical L17
  constraint coincident L9 L14.start
  constraint horizontal L18
  constraint vertical L19
  constraint horizontal L20
  constraint vertical L21
  constraint coincident L9 L18.start
  constraint horizontal L22
  constraint vertical L23
  constraint horizontal L24
  constraint vertical L25
  constraint coincident L9 L22.start
  constraint horizontal L26
  constraint vertical L27
  constraint horizontal L28
  constraint vertical L29
  constraint coincident L9 L26.start
  measures "d230" distance of L1 L8
  measures "d231" distance of L2 L6
  measures "d232" distance of L0 L5
  measures "d233" diameter of A0
  measures "d234" diameter of A1
  measures "d235" diameter of A2
  measures "d236" diameter of A3
  measures "d237" distance of L10.start L12.end
  measures "d238" distance of L1 L13
  measures "d239" distance of L11 L13
  measures "d240" distance of L14 L16
  measures "d241" distance of L11 L17
  measures "d242" distance of L15 L17
  measures "d243" distance of L18.start L18.end
  measures "d244" distance of L18.start L20.end
  measures "d245" distance of L15 L21
  measures "d246" distance of L22.start L22.end
  measures "d247" distance of L22.start L24.end
  measures "d248" distance of L19 L25
  measures "d249" distance of L26.start L26.end
  measures "d250" distance of L26.start L28.end
  measures "d251" distance of L23 L29
extrude "Extrude20" add sketch "IO Plate" against normal blind 1 from surface at -170 separate body contours L0 L1 L2 L9 L11 L12 L13 L15 L16 L17 L19 L20 L21 L23 L24 L25 L27 L28 L29 | L1 L2 L3 L9 L10 L14 L18 L22 L26 | L4 L5 L6 L7 L8 | A0 | A1 | A2 | A3 makes body 16
extrude "Extrude21" add sketch "IO Plate" against normal blind 16 from surface at -171 contours L4 L5 L6 L7 L8 | A0 | A1 | A2 | A3 bodies 16
extrude "Extrude22" cut sketch "IO Plate" along normal blind 3.8 from surface at -187 contours A0 | A1 | A2 | A3 bodies 16
extrude "Extrude23" cut sketch "Back Plate" along normal blind 6.3 from surface at -187 contours A6 | A7 | A8 | A9 bodies 16
extrude "Extrude24" cut 1 faces at (118.6833, -9.4333, -170) along direction (0, 0, -1) blind 0.2 on bodies 16 bodies 16
fillet "Fillet2" radius 2 4 edges at (63.8, 31, -178.6) (171.2, 31, -178.6) (63.8, -15, -178.6) (171.2, -15, -178.6) on bodies 16
component "Component" placed x (1, 0, 0) y (0, 1, 0) z (0, 0, 1) at (0, 0, 0)
equation "d42 = 80 mm + 15 mm + 3 mm + 1.7 mm + 3 mm"
named bodies: "Mini-ITX Board", "Base", "Leg", "Top", "IO Plate"
